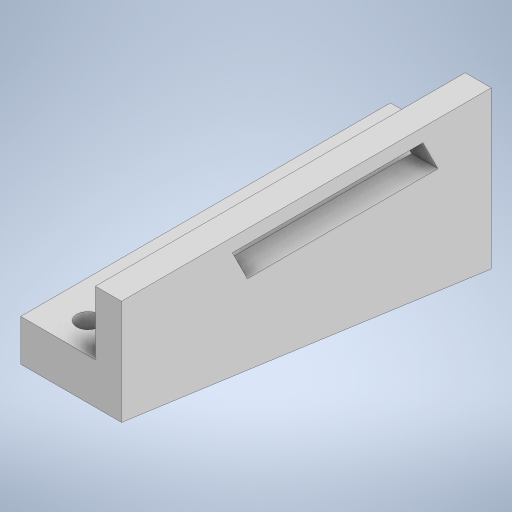
# Autodesk Inventor part: Podkladki_pod_laptopa
Saved by Autodesk Inventor 2024 (Build 280153000, 153)
## iProperties
Created: 2023-12-18
Part Number: Podkladki_pod_laptopa
Material: Generic
Document SubType Name: Modeling
Designer: Piter
Density: 1 g/cm^3
Appearance: Default
Author: Piter
Autodesk Inventor part; units mm, degrees
ref_plane "YZ Plane" through (0, 0, 0) normal (1, 0, 0) x (0, 1, 0)
ref_plane "XZ Plane" through (0, 0, 0) normal (0, 1, 0) x (-1, 0, 0)
ref_plane "XY Plane" through (0, 0, 0) normal (0, 0, 1) x (1, 0, 0)
sketch "Sketch1" plane through (0, 0, 0) normal (0, 1, 0) x (-1, 0, 0)
  line L0 (0, 0) -> (20, 0)
  line L1 (20, 0) -> (20, -99)
  line L2 (20, -99) -> (0, -99)
  line L3 (0, -99) -> (0, 0)
  line L4 (10, 0) -> (10, -8)
  circle A0 centre (10, -8) radius 3
  line L5 (10, -99) -> (10, -91)
  circle A1 centre (10, -91) radius 3
  line L6 (0, -99) -> (-7, -99)
  line L7 (-7, -99) -> (-7, 0)
  line L8 (-7, 0) -> (0, 0)
  line L9 (0, 0) -> (0, -99)
  dimension "d0" = 20
  dimension "d1" = 99
  dimension "d2" = 8
  dimension "d3" = 6
  dimension "d4" = 8
  dimension "d5" = 6
  dimension "d8" = 7
  constraints: 20 end point, 4 parallel, 2 centre point, 2 coincident, 2 horizontal, 2 midpoint, 2 perpendicular, 2 vertical
  measures "d0" distance of L1.end L2.end
  measures "d1" distance of L0.end L1.end
  measures "d2" distance of L4.start L4.end
  measures "d3" diameter of A0
  measures "d4" distance of L5.start L5.end
  measures "d5" diameter of A1
  measures "d8" distance of L7.end L8.end
extrude "Extrusion1" add sketch "Sketch1" along normal blind 25 contours L0 L1 L2 L3
extrude "Extrusion2" add sketch "Sketch1" along normal blind 42 contours L3 L6 L7 L8
sketch "Sketch2" plane through (0, 25, 0) normal (-1, 0, 0) x (0, 0, 1)
  line L0 (-84.6677, 5.4134) -> (-33.6677, 5.4134)
  line L1 (-33.6677, 5.4134) -> (-33.6677, 13.4134)
  line L2 (0, 17) -> (-99, 17) projected
  line L3 (-33.6677, 13.4134) -> (-29.6677, 13.4134)
  line L4 (-29.6677, 13.4134) -> (-80.6677, 13.4134)
  line L5 (-80.6677, 13.4134) -> (-84.6677, 5.4134)
  line L6 (-29.6677, 13.4134) -> (-33.6677, 5.4134)
  point P0 (0, -25)
  point P1 (-33.6677, 13.4134)
  dimension "d11" = 51
  dimension "d12" = 8
  dimension "d13" = 4
  dimension "d14" = 51
  constraints: 12 end point, 2 horizontal, 1 perpendicular, 1 point on line
  measures "d11" distance of L0.start L0.end
  measures "d12" distance of L0.end L1.end
  measures "d13" distance of L1.end L3.end
  measures "d14" distance of L3.end L4.end
extrude "Extrusion3" cut sketch "Sketch2" against normal through all
sketch "Sketch3" plane through (-20, 0, -99) normal (-1, 0, 0) x (0, 0, 1)
  line L0 (0, 0) -> (99, 13.9135)
  line L1 (99, 0) -> (99, 42) projected
  line L2 (0, 0) -> (99.9729, 0) construction
  line L3 (99, 13.9135) -> (99, 0)
  line L4 (99, 0) -> (0, 0)
  dimension "d17" = 8
  constraints: 8 end point, 1 collinear, 1 equal length, 1 horizontal, 1 perpendicular, 1 point on line
  measures "d17" angle of L2 L0
extrude "Extrusion4" cut sketch "Sketch3" against normal through all
body "Solid1"
